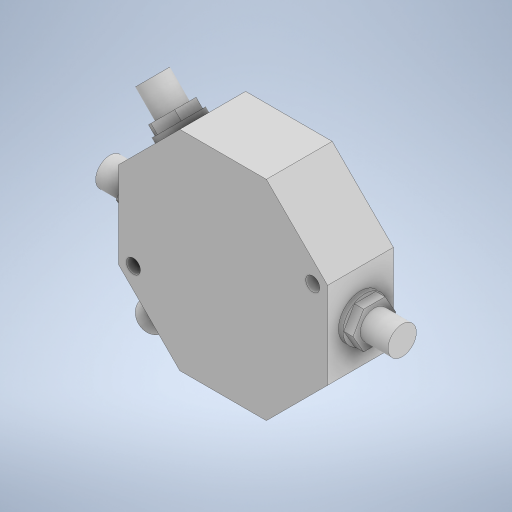
# Autodesk Inventor part: signal_combiner
Saved by Autodesk Inventor 2023 (Build 270158000, 158)
## iProperties
Created: 2023-05-29
Part Number: signal_combiner
Material: 一般
Document SubType Name: Modeling
Designer: 310611102
Density: 1 g/cm^3
Appearance: 預設
Author: 310611102
Autodesk Inventor part; units mm, degrees
ref_plane "YZ Plane" through (0, 0, 0) normal (1, 0, 0) x (0, 1, 0)
ref_plane "XZ Plane" through (0, 0, 0) normal (0, 1, 0) x (-1, 0, 0)
ref_plane "XY Plane" through (0, 0, 0) normal (0, 0, 1) x (1, 0, 0)
sketch "Sketch1" plane through (0, 0, 0) normal (0, 0, 1) x (1, 0, 0)
  line L0 (-22.55, 9.3405) -> (-9.3405, 22.55)
  line L1 (-9.3405, 22.55) -> (9.3405, 22.55)
  line L2 (9.3405, 22.55) -> (22.55, 9.3405)
  line L3 (22.55, 9.3405) -> (22.55, -9.3405)
  line L4 (22.55, -9.3405) -> (9.3405, -22.55)
  line L5 (9.3405, -22.55) -> (-9.3405, -22.55)
  line L6 (-9.3405, -22.55) -> (-22.55, -9.3405)
  line L7 (-22.55, -9.3405) -> (-22.55, 9.3405)
  point P0 (0, 0)
  point P1 (0, 0)
  point P2 (0, 22.55)
  dimension "d0" = 45.1
  constraints: 16 end point, 1 coincident, 1 midpoint, 1 vertical, 1 vertical alignment, 17 other
  measures "d0" distance between parallel lines of L3 L7
extrude "Extrusion1" add sketch "Sketch1" along normal blind 14.2
sketch "Sketch2" plane through (22.55, -9.3405, 0) normal (1, 0, 0) x (0, 0, -1)
  circle A0 centre (-7.1, 9.3405) radius 4.75
  line L0 (0, 0) -> (0, 18.681) projected
  line L1 (0, 18.681) -> (-14.2, 18.681) projected
  point P0 (0, 9.3405)
  point P1 (0, 9.3405)
  point P2 (-7.1, 18.681)
  dimension "d3" = 9.5
  constraints: 2 midpoint, 1 centre point, 1 horizontal alignment, 1 vertical alignment
  measures "d3" diameter of A0
extrude "Extrusion2" add sketch "Sketch2" along normal blind 1
sketch "Sketch3" plane through (23.55, 0, 7.1) normal (1, 0, 0) x (0, 0, -1)
  line L0 (4.6188, 0) -> (2.3094, -4)
  line L1 (2.3094, -4) -> (-2.3094, -4)
  line L2 (-2.3094, -4) -> (-4.6188, 0)
  line L3 (-4.6188, 0) -> (-2.3094, 4)
  line L4 (-2.3094, 4) -> (2.3094, 4)
  line L5 (2.3094, 4) -> (4.6188, 0)
  line L6 (7.1, 9.3405) -> (-7.1, 9.3405) projected
  point P0 (7.1, 0)
  point P1 (0, 0)
  point P2 (0, 9.3405)
  dimension "d6" = 8
  constraints: 12 end point, 2 horizontal alignment, 1 midpoint, 1 vertical alignment, 13 other
  measures "d6" distance between parallel lines of L2 L5
extrude "Extrusion3" add sketch "Sketch3" along normal blind 2
sketch "Sketch5" plane through (25.55, 0, 7.1) normal (1, 0, 0) x (0, 0, -1)
  circle A0 centre (0, 0) radius 3.05
  point P0 (7.1, 0)
  dimension "d9" = 6.1
  constraints: 1 centre point
  measures "d9" diameter of A0
extrude "Extrusion4" add sketch "Sketch5" along normal blind 6
pattern_circular "Circular Pattern1" count 2 over 135 about axis through (0, 0, -10) along (0, 0, 1) of "Extrusion2", "Extrusion3", "Extrusion4"
pattern_circular "Circular Pattern2" count 2 over 360 about axis through (0, 0, -10) along (0, 0, 1) of "Extrusion2", "Extrusion3", "Extrusion4"
pattern_circular "Circular Pattern3" count 2 over 225 about axis through (0, 0, -10) along (0, 0, 1) of "Extrusion2", "Extrusion3", "Extrusion4"
sketch "Sketch7" plane through (0, 0, 14.2) normal (0, 0, 1) x (1, 0, 0)
  circle A0 centre (19.35, 8.015) radius 1.5
  line L0 (22.55, 9.3405) -> (9.3405, 22.55) projected
  line L1 (22.55, 9.3405) -> (-22.55, -9.3405)
  circle A1 centre (-19.35, -8.015) radius 1.5
  point P0 (0, 0)
  dimension "d21" = 3
  dimension "d22" = 6.4
  dimension "d25" = 360
  constraints: 2 centre point, 2 end point, 1 point on line, 5 other
  measures "d21" diameter of A0
  measures "d22" diameter of A0.centre L0
extrude "Extrusion5" cut sketch "Sketch7" against normal through all
body "Solid1"
